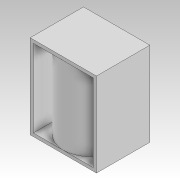
# Autodesk Inventor part: Solenoid
Saved by Autodesk Inventor 2020 (Build 240168000, 168)
## iProperties
Created: 2021-08-03
Part Number: Solenoid
Material: Generic
Document SubType Name: Modeling
Designer: DDeGo
Density: 1 g/cm^3
Appearance: Default
Author: DDeGo
Autodesk Inventor part; units mm, degrees
ref_plane "YZ Plane" through (0, 0, 0) normal (1, 0, 0) x (0, 1, 0)
ref_plane "XZ Plane" through (0, 0, 0) normal (0, 1, 0) x (-1, 0, 0)
ref_plane "XY Plane" through (0, 0, 0) normal (0, 0, 1) x (1, 0, 0)
sketch "Sketch1" plane through (0, 0, 0) normal (0, 0, 1) x (1, 0, 0)
  line L0 (-10.25, -13) -> (10.25, -13)
  line L1 (10.25, -13) -> (10.25, 13)
  line L2 (10.25, 13) -> (-10.25, 13)
  line L3 (-10.25, 13) -> (-10.25, -13)
  line L4 (-10.25, -13) -> (10.25, 13) construction
  line L5 (10.25, -13) -> (-10.25, 13) construction
  line L6 (-9.25, 12) -> (9.25, 12)
  line L7 (9.25, 12) -> (9.25, -12)
  line L8 (9.25, -12) -> (-9.25, -12)
  line L9 (-9.25, -12) -> (-9.25, 12)
  point P0 (0, 0)
  dimension "d0" = 26
  dimension "d1" = 20.5
  dimension "d2" = 1
  constraints: 20 end point, 4 parallel, 2 midpoint, 2 perpendicular, 1 horizontal, 3 other
  measures "d0" distance of L0.end L1.end
  measures "d1" distance of L1.end L2.end
  measures "d2" distance between parallel lines of L2 L6
extrude "Extrusion1" add sketch "Sketch1" along normal blind 16.5
sketch "Sketch2" plane through (-9.25, -12, 0) normal (0, 1, 0) x (1, 0, 0)
  line L0 (0, -16.5) -> (18.5, 0) construction
  circle A0 centre (9.25, -8.25) radius 8.25
  point P0 (9.25, 0)
  constraints: 2 end point, 1 midpoint, 1 vertical alignment, 2 other
extrude "Extrusion2" add sketch "Sketch2" along normal up to surface (24 mm away)
sketch "Sketch6" plane through (-10.25, -13, 0) normal (0, -1, 0) x (1, 0, 0)
  arc A0 (10.25, 0) -> (10.25, 16.5) centre (10.25, 8.25) ccw projected
  arc A1 (10.25, 16.5) -> (10.25, 0) centre (10.25, 8.25) ccw projected
  arc A2 (10.25, 16.5) -> (10.25, 0) centre (10.25, 8.25) ccw projected
  arc A3 (10.25, 0) -> (10.25, 16.5) centre (10.25, 8.25) ccw projected
  arc A4 (10.25, 16.5) -> (10.25, 0) centre (10.25, 8.25) ccw projected
  circle A5 centre (10.25, 8.25) radius 3.9566
  constraints: 1 centre point, 1 coincident
extrude "Extrusion6" cut sketch "Sketch6" against normal blind 10 contours A5
sketch "Sketch3" plane through (-10.25, -13, 0) normal (0, -1, 0) x (1, 0, 0)
  line L0 (0, 0) -> (0, 16.5) construction
  line L1 (0, 16.5) -> (20.5, 16.5) construction
  line L2 (0, 0) -> (20.5, 16.5) construction
  line L3 (10.25, 16.5) -> (1, 16.5) projected
  line L4 (18.5, 0) -> (2, 0)
  line L5 (2, 0) -> (2, 16.5)
  line L6 (2, 16.5) -> (18.5, 16.5)
  line L7 (18.5, 16.5) -> (18.5, 0)
  line L8 (18.5, 0) -> (2, 16.5) construction
  line L9 (2, 0) -> (18.5, 16.5) construction
  point P0 (10.25, 0)
  point P1 (10.25, 8.25)
  dimension "d7" = 16.5
  constraints: 14 end point, 3 midpoint, 2 parallel, 1 horizontal, 1 perpendicular, 1 point on line
  measures "d7" distance between parallel lines of L7 L5
sketch "Sketch4" plane through (0, 0, 16.5) normal (0, 0, 1) x (1, 0, 0)
  line L0 (-8.25, -13) -> (-8.25, -27) construction
  line L1 (-8.25, -27) -> (8.25, -27) construction
  line L2 (-8.25, -13) -> (8.25, -27) construction
  circle A0 centre (0, -20) radius 2.25
  circle A1 centre (0, -20) radius 1.75
  point P0 (0, 0)
  dimension "d10" = 4.5
  dimension "d11" = 0.5
  constraints: 2 centre point, 2 end point, 1 coincident, 1 midpoint
  measures "d10" diameter of A0
  measures "d11" radial gap between concentric circles of A0 A1
sketch "Sketch5" plane through (-10.25, -27, 0) normal (0, -1, 0) x (1, 0, 0)
  line L0 (2, 16.5) -> (2, 0) construction
  line L1 (18.5, 0) -> (18.5, 16.5) construction
  line L2 (2, 0) -> (18.5, 16.5) construction
  circle A0 centre (10.25, 8.25) radius 2.25
  circle A1 centre (10.25, 8.25) radius 1.75
  point P0 (10.25, 0)
  dimension "d14" = 4.5
  dimension "d15" = 0.5
  constraints: 2 centre point, 2 end point, 1 coincident, 1 midpoint
  measures "d14" diameter of A0
  measures "d15" radial gap between concentric circles of A0 A1
body "Solid1"
